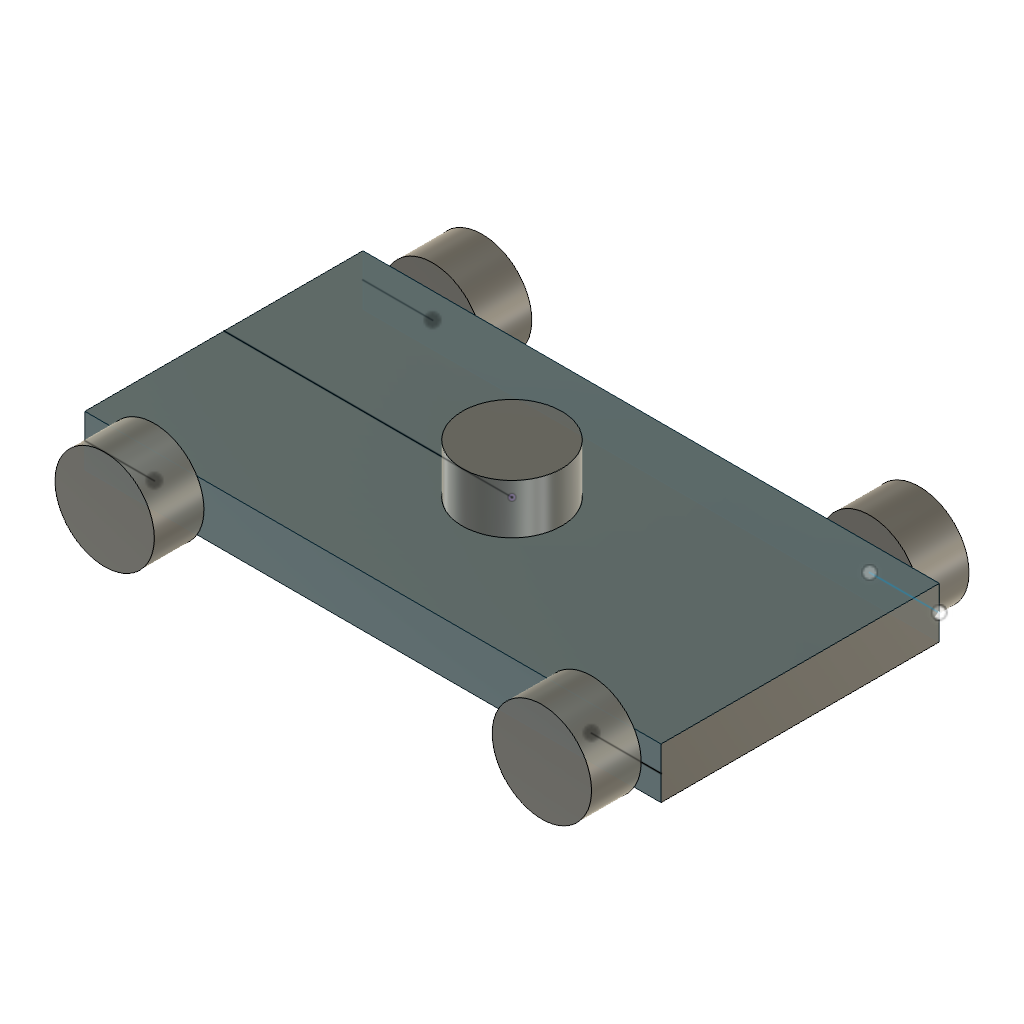
eternal_bot_minimal (Autodesk Fusion 360 design; units mm, degrees)
part number: 2026-10-06-23-32-50-978
part number: 2026-10-06-23-51-29-905
part number: 2026-10-06-23-51-29-913
part number: 2026-10-06-23-51-29-915
part number: 2026-10-06-23-51-29-918
part number: 2026-10-06-23-51-29-920
part number: 2026-10-06-23-51-29-922
part number: 2026-10-07-01-17-49-263
part number: 2026-10-07-01-17-49-318
part number: 2026-10-07-01-17-49-330
part number: 2026-10-07-01-17-49-341
part number: 2026-10-07-01-17-49-352
part number: 2026-10-07-01-17-49-363
Autodesk Fusion 360 part; units mm, degrees
sketch "Sketch1" plane through (0, 0, 0) normal (0, 0, 1) x (1, 0, 0)
  line L0 (290, 140) -> (-290, 140)
  line L1 (-290, 140) -> (-290, -140)
  line L2 (-290, -140) -> (290, -140)
  line L3 (290, -140) -> (290, 140)
  line L4 (290, 140) -> (-290, -140) construction
  line L5 (-290, 140) -> (290, -140) construction
  dimension "d1" = 580
  dimension "d2" = 280
  constraint horizontal L0
  constraint perpendicular L0 L1
  constraint parallel L0 L2
  constraint parallel L1 L3
  constraint coincident L4 origin
  constraint coincident L5 origin
  measures "d1" distance of L1.end L2.end
  measures "d2" distance of L0.end L1.end
extrude "Extrude1" add sketch "Sketch1" along normal blind 51.2 makes body 1
sketch "Sketch2" plane through (0, -140, 0) normal (0, -1, 0) x (1, 0, 0)
  line L0 (-290, 0) -> (290, 0)
  line L1 (290, 0) -> (290, 51.2)
  line L2 (290, 51.2) -> (-290, 51.2)
  line L3 (-290, 51.2) -> (-290, 0)
  line L4 (290, 25.6) -> (220, 25.6)
  circle A0 centre (220, 25.6) radius 50
  dimension "d5" = 70
  dimension "d6" = 100
  constraint midpoint L1 L4.start
  constraint perpendicular L1 L4
  constraint coincident L4.end A0.centre
  measures "d5" distance of L4.start L4.end
  measures "d6" diameter of A0
extrude "Extrude2" add sketch "Sketch2" along normal blind 50 separate body contours L0 L2 A0 | L0 A0 | L2 A0 makes body 2
sketch "Sketch3" plane through (0, 0, 51.2) normal (0, 0, 1) x (-1, 0, 0)
  line L0 (-290, 140) -> (-290, -140)
  line L1 (-290, -140) -> (290, -140)
  line L2 (290, -140) -> (290, 140)
  line L3 (290, 140) -> (-290, 140)
  line L4 (0, 0) -> (290, 0)
  constraint coincident L4.start origin
  constraint midpoint L2 L4.end
mirror "Mirror1" about plane through (0, 0, 0) normal (0, 1, 0) of bodies 2 makes body 3
mirror "Mirror2" about plane through (0, 0, 0) normal (1, 0, 0) of bodies 3 2 makes body 4 at (-224.8492, -140, 50.3967) makes body 5 at (-224.8492, 140, 50.3967)
sketch "Sketch4" plane through (0, 0, 51.2) normal (0, 0, 1) x (-1, 0, 0)
  circle A0 centre (0, 0) radius 50
  dimension "d13" = 100
  constraint coincident A0.centre origin
  measures "d13" diameter of A0
extrude "Extrude3" add sketch "Sketch4" along normal blind 50 separate body makes body 6
copy_body "Body->Comp1" bodies 1 removing the originals makes body 7 in component "old_component"
copy_body "Body->Comp2" bodies 2 removing the originals makes body 8 in component "old_component (1)"
copy_body "Body->Comp3" bodies 3 removing the originals makes body 9 in component "old_component (2)"
copy_body "Body->Comp4" bodies 4 removing the originals makes body 10 in component "old_component (3)"
copy_body "Body->Comp5" bodies 5 removing the originals makes body 11 in component "old_component (4)"
copy_body "Body->Comp6" bodies 6 removing the originals makes body 12 in component "old_component (5)"
sketch "Sketch5" plane through (0, 140, 0) normal (0, 1, 0) x (-1, 0, 0)
  line L0 (-290, 0) -> (290, 0)
  line L1 (290, 0) -> (290, 51.2)
  line L2 (290, 51.2) -> (-290, 51.2)
  line L3 (-290, 51.2) -> (-290, 0)
  line L4 (-290, 25.6) -> (-220, 25.6)
  line L5 (290, 25.6) -> (220, 25.6)
  dimension "d16" = 70
  dimension "d31" = 70
  constraint perpendicular L3 L4
  constraint midpoint L1 L5.start
  constraint perpendicular L1 L5
  measures "d16" distance of L4.start L4.end
  measures "d31" distance of L5.start L5.end
sketch "Sketch6" plane through (0, -140, 0) normal (0, -1, 0) x (1, 0, 0)
  line L0 (-290, 0) -> (290, 0)
  line L1 (290, 0) -> (290, 51.2)
  line L2 (290, 51.2) -> (-290, 51.2)
  line L3 (-290, 51.2) -> (-290, 0)
  line L4 (290, 25.6) -> (220, 25.6)
  line L5 (-290, 25.6) -> (-220, 25.6)
  dimension "d21" = 70
  dimension "d22" = 70
  constraint midpoint L1 L4.start
  constraint perpendicular L1 L4
  constraint midpoint L3 L5.start
  constraint perpendicular L3 L5
  measures "d21" distance of L4.start L4.end
  measures "d22" distance of L5.start L5.end
copy_body "CopyPasteBodies1" bodies 7 makes body 13 in component "base_link"
copy_body "CopyPasteBodies1'" bodies 8 makes body 14 in component "front_right_1"
copy_body "CopyPasteBodies1''" bodies 9 makes body 15 in component "front_left_1"
copy_body "CopyPasteBodies1'''" bodies 10 makes body 16 in component "rear_right_1"
copy_body "CopyPasteBodies1''''" bodies 11 makes body 17 in component "rear_left_1"
copy_body "CopyPasteBodies1'''''" bodies 12 makes body 18 in component "lidar_1"
component "old_component" placed x (1, 0, 0) y (0, 1, 0) z (0, 0, 1) at (0, 0, 0)
component "old_component (1)" placed x (1, 0, 0) y (0, 1, 0) z (0, 0, 1) at (0, 0, 0)
component "old_component (2)" placed x (1, 0, 0) y (0, 1, 0) z (0, 0, 1) at (0, 0, 0)
component "old_component (3)" placed x (1, 0, 0) y (0, 1, 0) z (0, 0, 1) at (0, 0, 0)
component "old_component (4)" placed x (1, 0, 0) y (0, 1, 0) z (0, 0, 1) at (0, 0, 0)
component "old_component (5)" placed x (1, 0, 0) y (0, 1, 0) z (0, 0, 1) at (0, 0, 0)
component "base_link" placed x (1, 0, 0) y (0, 1, 0) z (0, 0, 1) at (0, 0, 0)
component "front_right_1" placed x (1, 0, 0) y (0, 1, 0) z (0, 0, 1) at (0, 0, 0)
component "front_left_1" placed x (1, 0, 0) y (0, 1, 0) z (0, 0, 1) at (0, 0, 0)
component "rear_right_1" placed x (1, 0, 0) y (0, 1, 0) z (0, 0, 1) at (0, 0, 0)
component "rear_left_1" placed x (1, 0, 0) y (0, 1, 0) z (0, 0, 1) at (0, 0, 0)
component "lidar_1" placed x (1, 0, 0) y (0, 1, 0) z (0, 0, 1) at (0, 0, 0)
named bodies: "base_link", "front_right", "front_left", "rear_right", "rear_left", "lidar"
